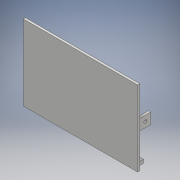
# Autodesk Inventor part: Encaixe
Saved by Autodesk Inventor 2018 (Build 220112000, 112)
## iProperties
Created: 2018-05-04
Part Number: Encaixe
Material: Genérico
Document SubType Name: Modeling
Designer: mirre
Density: 1 g/cm^3
Appearance: Padrão
Author: mirre
Autodesk Inventor part; units mm, degrees
ref_plane "YZ Plane" through (0, 0, 0) normal (1, 0, 0) x (0, 1, 0)
sketch "Esboço6" plane through (0, 0, 0) normal (0, 1, 0) x (-1, 0, 0)
  line L0 (0, 0) -> (156, 0)
  line L1 (156, 0) -> (156, -103)
  line L2 (156, -103) -> (0, -103)
  line L3 (0, -103) -> (0, 0)
  dimension "d22" = 156
  dimension "d23" = 103
  constraints: 8 end point, 2 parallel, 1 horizontal, 1 perpendicular
  measures "d22" distance of L1.end L2.end
  measures "d23" distance between parallel lines of L2 L0
extrude "Extrusão4" add sketch "Esboço6" along normal blind 3
sketch "Esboço7" plane through (0, 3, 0) normal (0, 1, 0) x (1, 0, 0)
  line L0 (-152.9, 99.9) -> (-3.1, 99.9)
  line L1 (-3.1, 99.9) -> (-3.1, 3.1)
  line L2 (-3.1, 3.1) -> (-152.9, 3.1)
  line L3 (-152.9, 3.1) -> (-152.9, 99.9)
  line L4 (0, 0) -> (0, 103) projected
  line L5 (0, 103) -> (-156, 103) projected
  line L6 (-156, 103) -> (-156, 0) projected
  line L7 (-156, 0) -> (0, 0) projected
  line L8 (-149.9, 96.9) -> (-6.1, 96.9)
  line L9 (-6.1, 96.9) -> (-6.1, 6.1)
  line L10 (-6.1, 6.1) -> (-149.9, 6.1)
  line L11 (-149.9, 6.1) -> (-149.9, 96.9)
  dimension "d26" = 3.1
  dimension "d27" = 3.1
  dimension "d28" = 3.1
  dimension "d29" = 3.1
  dimension "d30" = 3
  dimension "d31" = 3
  dimension "d32" = 3
  dimension "d33" = 3
  constraints: 16 end point, 4 parallel, 2 horizontal, 2 perpendicular
  measures "d26" distance between parallel lines of L4 L1
  measures "d27" distance between parallel lines of L5 L0
  measures "d28" distance between parallel lines of L6 L3
  measures "d29" distance between parallel lines of L7 L2
  measures "d30" distance between parallel lines of L0 L8
  measures "d31" distance between parallel lines of L1 L9
  measures "d32" distance between parallel lines of L10 L2
  measures "d33" distance between parallel lines of L11 L3
extrude "Extrusão5" add sketch "Esboço7" along normal blind 3 contours L0 L1 L2 L3
sketch "Esboço10" plane through (0, 6, 0) normal (0, 1, 0) x (1, 0, 0)
  line L0 (-3.1, 99.9) -> (-3.1, 3.1) projected
  line L1 (-3.1, 99.9) -> (-8.1, 99.9)
  line L2 (-8.1, 99.9) -> (-8.1, 94.9)
  line L3 (-8.1, 94.9) -> (-3.1, 94.9)
  line L4 (-3.1, 94.9) -> (-3.1, 99.9)
  line L5 (-152.9, 99.9) -> (-3.1, 99.9) projected
  line L6 (-93.1, 99.9) -> (-101.1, 99.9)
  line L7 (-101.1, 99.9) -> (-101.1, 94.9)
  line L8 (-101.1, 94.9) -> (-93.1, 94.9)
  line L9 (-93.1, 94.9) -> (-93.1, 99.9)
  point P0 (0, 0)
  dimension "d36" = 5
  dimension "d37" = 5
  dimension "d38" = 85
  dimension "d39" = 8
  dimension "d40" = 5
  constraints: 16 end point, 4 parallel, 2 horizontal, 2 perpendicular, 1 point on line
  measures "d36" distance of L3.end L2.end
  measures "d37" distance between parallel lines of L1 L3
  measures "d38" distance between parallel lines of L9 L2
  measures "d39" distance between parallel lines of L7 L9
  measures "d40" distance between parallel lines of L8 L5
extrude "Extrusão6" add sketch "Esboço10" along normal blind 5 and the other way blind 6
sketch "Esboço13" plane through (-101.1, 3, -94.9) normal (0, 0, 1) x (1, 0, 0)
  line L0 (93, 3) -> (8, 3) projected
  line L1 (8, 3) -> (0, 3)
  line L2 (0, 3) -> (0, 23)
  line L3 (0, 23) -> (3, 23)
  line L4 (3, 23) -> (3, 8)
  line L5 (8, 8) -> (0, 8) projected
  line L6 (3, 8) -> (8, 8)
  line L7 (8, 8) -> (8, 3)
  point P0 (101.1, -3)
  dimension "d45" = 8
  dimension "d46" = 20
  dimension "d47" = 3
  constraints: 12 end point, 3 perpendicular, 2 collinear, 1 vertical
  measures "d45" distance of L0.end L1.end
  measures "d46" distance between parallel lines of L3 L1
  measures "d47" distance between parallel lines of L4 L2
extrude "Extrusão7" add sketch "Esboço13" against normal blind 5 contours L2 L3 L4 L5
sketch "Esboço14" plane through (-101.1, 3, -94.9) normal (0, 0, 1) x (1, 0, 0)
  line L0 (0, 3) -> (0, 23) projected
  line L1 (0, 23) -> (3, 23) projected
  line L2 (0, 23) -> (3, 23)
  line L3 (-54.9, -3) -> (101.1, -3) projected
  line L4 (0, 0) -> (0, 23)
  line L5 (0, 0) -> (8, 0)
  line L6 (-51.8, 0) -> (98, 0) projected
  line L7 (8, 0) -> (8, 3)
  line L8 (93, 3) -> (8, 3) projected
  line L9 (8, 3) -> (3, 3)
  line L10 (3, 3) -> (3, 23)
  line L11 (3, 23) -> (3, 8) projected
  line L12 (8, 8) -> (3, 8) projected
  dimension "d53" = 8
  dimension "d54" = 5
  dimension "d55" = 5
  constraints: 12 end point, 3 collinear, 2 perpendicular, 1 point on line
  measures "d53" distance of L4.start L5.end
  measures "d54" distance between parallel lines of L12 L9
  measures "d55" distance between parallel lines of L7 L10
extrude "Extrusão8" add sketch "Esboço14" along normal blind 2
ref_plane "Plano de trabalho1" through (-6.1, 6, -50.5) normal (-1, 0, 0) x (0, 0, 1)
ref_plane "Plano de trabalho2" through (-149.9, 6, -51.5) normal (1, 0, 0) x (0, 0, -1)
sketch "Esboço18" plane through (-6.1, 6, -50.5) normal (-1, 0, 0) x (0, 0, 1)
  line L0 (6.5, 0) -> (-8.5, 0)
  line L1 (-8.5, 0) -> (-8.5, 15)
  line L2 (-8.5, 15) -> (6.5, 15)
  line L3 (6.5, 15) -> (6.5, 0)
  line L4 (-49.4, 0) -> (47.4, 0) projected
  line L5 (47.4, -3) -> (47.4, 0) projected
  dimension "d67" = 15
  dimension "d68" = 15
  dimension "d71" = 40.9
  constraints: 8 end point, 2 collinear, 1 horizontal, 1 parallel
  measures "d67" distance between parallel lines of L2 L0
  measures "d68" distance between parallel lines of L1 L3
  measures "d71" distance between parallel lines of L5 L3
extrude "Extrusão9" add sketch "Esboço18" against normal blind 3
sketch "Esboço19" plane through (-149.9, 6, -51.5) normal (1, 0, 0) x (0, 0, -1)
  line L0 (-7.5, 0) -> (7.5, 0)
  line L1 (7.5, 0) -> (7.5, 15)
  line L2 (7.5, 15) -> (-7.5, 15)
  line L3 (-7.5, 15) -> (-7.5, 0)
  line L4 (48.4, -3) -> (48.4, 0) projected
  line L5 (48.4, 0) -> (-48.4, 0) projected
  point P0 (-51.5, -6)
  dimension "d72" = 15
  dimension "d73" = 15
  dimension "d74" = 40.9
  constraints: 8 end point, 2 parallel, 1 collinear, 1 horizontal, 1 perpendicular
  measures "d72" distance of L2.end L1.end
  measures "d73" distance between parallel lines of L2 L0
  measures "d74" distance between parallel lines of L4 L1
extrude "Extrusão10" add sketch "Esboço19" against normal blind 3
sketch "Esboço21" plane through (-152.9, 3, -99.9) normal (-1, 0, 0) x (0, 0, 1)
  circle A0 centre (48.4, 10.5) radius 2.05
  line L0 (55.9, 3) -> (55.9, 18) projected
  line L1 (55.9, 18) -> (40.9, 18) projected
  dimension "d87" = 7.5
  dimension "d88" = 7.5
  dimension "d89" = 4.1
  constraints: 1 centre point
  measures "d87" distance from line of L0 A0.centre
  measures "d88" distance from line of L1 A0.centre
  measures "d89" diameter of A0
extrude "Extrusão13" cut sketch "Esboço21" against normal through all
sketch "Esboço22" plane through (-152.9, 3, -99.9) normal (-1, 0, 0) x (0, 0, 1)
  line L0 (5, 3) -> (40.9, 3) projected
  line L1 (99.9, 0) -> (-3.1, 0) projected
  line L2 (5.9, 3) -> (3.9, 3)
  line L3 (3.9, 3) -> (3.9, 0)
  line L4 (3.9, 0) -> (5.9, 0)
  line L5 (5.9, 0) -> (5.9, 3)
  line L6 (-3.1, -3) -> (-3.1, 0) projected
  dimension "d92" = 2
  dimension "d93" = 7
  constraints: 8 end point, 2 parallel, 2 point on line, 1 horizontal, 1 perpendicular
  measures "d92" distance between parallel lines of L5 L3
  measures "d93" distance between parallel lines of L6 L3
extrude "Extrusão14" cut sketch "Esboço22" against normal blind 10
